Autodesk Inventor part; units mm, degrees
(part 9 of 13)
  line L3844 (34.289, 23.3701) -> (34.289, 23.1233) construction
  line L3845 (34.289, 23.1233) -> (34.4891, 22.9231) construction
  line L3846 (34.4891, 22.9231) -> (34.7358, 22.9231) construction
  spline S1207 degree 3 poles (34.7358, 22.9231) (34.9826, 22.9231) (35.1829, 23.1233) (35.1829, 23.3701) knots 0 0 0 0 1 1 1 1
  line L3847 (34.7358, 22.9231) -> (34.9826, 22.9231) construction
  line L3848 (34.9826, 22.9231) -> (35.1829, 23.1233) construction
  line L3849 (35.1829, 23.1233) -> (35.1829, 23.3701) construction
  spline S1208 degree 3 poles (35.1829, 25.9242) (35.1829, 26.171) (34.9826, 26.3711) (34.7358, 26.3711) knots 0 0 0 0 1 1 1 1
  line L3850 (35.1829, 25.9242) -> (35.1829, 26.171) construction
  line L3851 (35.1829, 26.171) -> (34.9826, 26.3711) construction
  line L3852 (34.9826, 26.3711) -> (34.7358, 26.3711) construction
  spline S1209 degree 3 poles (34.7358, 26.3711) (34.4891, 26.3711) (34.289, 26.171) (34.289, 25.9242) knots 0 0 0 0 1 1 1 1
  line L3853 (34.7358, 26.3711) -> (34.4891, 26.3711) construction
  line L3854 (34.4891, 26.3711) -> (34.289, 26.171) construction
  line L3855 (34.289, 26.171) -> (34.289, 25.9242) construction
  spline S1210 degree 3 poles (34.289, 25.9242) (34.289, 25.6775) (34.4891, 25.4772) (34.7358, 25.4772) knots 0 0 0 0 1 1 1 1
  line L3856 (34.289, 25.9242) -> (34.289, 25.6775) construction
  line L3857 (34.289, 25.6775) -> (34.4891, 25.4772) construction
  line L3858 (34.4891, 25.4772) -> (34.7358, 25.4772) construction
  spline S1211 degree 3 poles (34.7358, 25.4772) (34.9826, 25.4772) (35.1829, 25.6775) (35.1829, 25.9242) knots 0 0 0 0 1 1 1 1
  line L3859 (34.7358, 25.4772) -> (34.9826, 25.4772) construction
  line L3860 (34.9826, 25.4772) -> (35.1829, 25.6775) construction
  line L3861 (35.1829, 25.6775) -> (35.1829, 25.9242) construction
  spline S1212 degree 3 poles (35.1829, 28.4784) (35.1829, 28.7251) (34.9826, 28.9252) (34.7358, 28.9252) knots 0 0 0 0 1 1 1 1
  line L3862 (35.1829, 28.4784) -> (35.1829, 28.7251) construction
  line L3863 (35.1829, 28.7251) -> (34.9826, 28.9252) construction
  line L3864 (34.9826, 28.9252) -> (34.7358, 28.9252) construction
  spline S1213 degree 3 poles (34.7358, 28.9252) (34.4891, 28.9252) (34.289, 28.7251) (34.289, 28.4784) knots 0 0 0 0 1 1 1 1
  line L3865 (34.7358, 28.9252) -> (34.4891, 28.9252) construction
  line L3866 (34.4891, 28.9252) -> (34.289, 28.7251) construction
  line L3867 (34.289, 28.7251) -> (34.289, 28.4784) construction
  spline S1214 degree 3 poles (34.289, 28.4784) (34.289, 28.2316) (34.4891, 28.0313) (34.7358, 28.0313) knots 0 0 0 0 1 1 1 1
  line L3868 (34.289, 28.4784) -> (34.289, 28.2316) construction
  line L3869 (34.289, 28.2316) -> (34.4891, 28.0313) construction
  line L3870 (34.4891, 28.0313) -> (34.7358, 28.0313) construction
  spline S1215 degree 3 poles (34.7358, 28.0313) (34.9826, 28.0313) (35.1829, 28.2316) (35.1829, 28.4784) knots 0 0 0 0 1 1 1 1
  line L3871 (34.7358, 28.0313) -> (34.9826, 28.0313) construction
  line L3872 (34.9826, 28.0313) -> (35.1829, 28.2316) construction
  line L3873 (35.1829, 28.2316) -> (35.1829, 28.4784) construction
  spline S1216 degree 3 poles (35.1829, 31.0325) (35.1829, 31.2793) (34.9826, 31.4793) (34.7358, 31.4793) knots 0 0 0 0 1 1 1 1
  line L3874 (35.1829, 31.0325) -> (35.1829, 31.2793) construction
  line L3875 (35.1829, 31.2793) -> (34.9826, 31.4793) construction
  line L3876 (34.9826, 31.4793) -> (34.7358, 31.4793) construction
  spline S1217 degree 3 poles (34.7358, 31.4793) (34.4891, 31.4793) (34.289, 31.2793) (34.289, 31.0325) knots 0 0 0 0 1 1 1 1
  line L3877 (34.7358, 31.4793) -> (34.4891, 31.4793) construction
  line L3878 (34.4891, 31.4793) -> (34.289, 31.2793) construction
  line L3879 (34.289, 31.2793) -> (34.289, 31.0325) construction
  spline S1218 degree 3 poles (34.289, 31.0325) (34.289, 30.7857) (34.4891, 30.5854) (34.7358, 30.5854) knots 0 0 0 0 1 1 1 1
  line L3880 (34.289, 31.0325) -> (34.289, 30.7857) construction
  line L3881 (34.289, 30.7857) -> (34.4891, 30.5854) construction
  line L3882 (34.4891, 30.5854) -> (34.7358, 30.5854) construction
  spline S1219 degree 3 poles (34.7358, 30.5854) (34.9826, 30.5854) (35.1829, 30.7857) (35.1829, 31.0325) knots 0 0 0 0 1 1 1 1
  line L3883 (34.7358, 30.5854) -> (34.9826, 30.5854) construction
  line L3884 (34.9826, 30.5854) -> (35.1829, 30.7857) construction
  line L3885 (35.1829, 30.7857) -> (35.1829, 31.0325) construction
  spline S1220 degree 3 poles (37.737, 20.816) (37.737, 21.0628) (37.5369, 21.2629) (37.29, 21.2629) knots 0 0 0 0 1 1 1 1
  line L3886 (37.737, 20.816) -> (37.737, 21.0628) construction
  line L3887 (37.737, 21.0628) -> (37.5369, 21.2629) construction
  line L3888 (37.5369, 21.2629) -> (37.29, 21.2629) construction
  spline S1221 degree 3 poles (37.29, 21.2629) (37.0431, 21.2629) (36.843, 21.0628) (36.843, 20.816) knots 0 0 0 0 1 1 1 1
  line L3889 (37.29, 21.2629) -> (37.0431, 21.2629) construction
  line L3890 (37.0431, 21.2629) -> (36.843, 21.0628) construction
  line L3891 (36.843, 21.0628) -> (36.843, 20.816) construction
  spline S1222 degree 3 poles (36.843, 20.816) (36.843, 20.5692) (37.0431, 20.369) (37.29, 20.369) knots 0 0 0 0 1 1 1 1
  line L3892 (36.843, 20.816) -> (36.843, 20.5692) construction
  line L3893 (36.843, 20.5692) -> (37.0431, 20.369) construction
  line L3894 (37.0431, 20.369) -> (37.29, 20.369) construction
  spline S1223 degree 3 poles (37.29, 20.369) (37.5369, 20.369) (37.737, 20.5692) (37.737, 20.816) knots 0 0 0 0 1 1 1 1
  line L3895 (37.29, 20.369) -> (37.5369, 20.369) construction
  line L3896 (37.5369, 20.369) -> (37.737, 20.5692) construction
  line L3897 (37.737, 20.5692) -> (37.737, 20.816) construction
  spline S1224 degree 3 poles (37.737, 23.3701) (37.737, 23.6169) (37.5369, 23.817) (37.29, 23.817) knots 0 0 0 0 1 1 1 1
  line L3898 (37.737, 23.3701) -> (37.737, 23.6169) construction
  line L3899 (37.737, 23.6169) -> (37.5369, 23.817) construction
  line L3900 (37.5369, 23.817) -> (37.29, 23.817) construction
  spline S1225 degree 3 poles (37.29, 23.817) (37.0431, 23.817) (36.843, 23.6169) (36.843, 23.3701) knots 0 0 0 0 1 1 1 1
  line L3901 (37.29, 23.817) -> (37.0431, 23.817) construction
  line L3902 (37.0431, 23.817) -> (36.843, 23.6169) construction
  line L3903 (36.843, 23.6169) -> (36.843, 23.3701) construction
  spline S1226 degree 3 poles (36.843, 23.3701) (36.843, 23.1233) (37.0431, 22.9231) (37.29, 22.9231) knots 0 0 0 0 1 1 1 1
  line L3904 (36.843, 23.3701) -> (36.843, 23.1233) construction
  line L3905 (36.843, 23.1233) -> (37.0431, 22.9231) construction
  line L3906 (37.0431, 22.9231) -> (37.29, 22.9231) construction
  spline S1227 degree 3 poles (37.29, 22.9231) (37.5369, 22.9231) (37.737, 23.1233) (37.737, 23.3701) knots 0 0 0 0 1 1 1 1
  line L3907 (37.29, 22.9231) -> (37.5369, 22.9231) construction
  line L3908 (37.5369, 22.9231) -> (37.737, 23.1233) construction
  line L3909 (37.737, 23.1233) -> (37.737, 23.3701) construction
  spline S1228 degree 3 poles (37.737, 25.9242) (37.737, 26.171) (37.5369, 26.3711) (37.29, 26.3711) knots 0 0 0 0 1 1 1 1
  line L3910 (37.737, 25.9242) -> (37.737, 26.171) construction
  line L3911 (37.737, 26.171) -> (37.5369, 26.3711) construction
  line L3912 (37.5369, 26.3711) -> (37.29, 26.3711) construction
  spline S1229 degree 3 poles (37.29, 26.3711) (37.0431, 26.3711) (36.843, 26.171) (36.843, 25.9242) knots 0 0 0 0 1 1 1 1
  line L3913 (37.29, 26.3711) -> (37.0431, 26.3711) construction
  line L3914 (37.0431, 26.3711) -> (36.843, 26.171) construction
  line L3915 (36.843, 26.171) -> (36.843, 25.9242) construction
  spline S1230 degree 3 poles (36.843, 25.9242) (36.843, 25.6775) (37.0431, 25.4772) (37.29, 25.4772) knots 0 0 0 0 1 1 1 1
  line L3916 (36.843, 25.9242) -> (36.843, 25.6775) construction
  line L3917 (36.843, 25.6775) -> (37.0431, 25.4772) construction
  line L3918 (37.0431, 25.4772) -> (37.29, 25.4772) construction
  spline S1231 degree 3 poles (37.29, 25.4772) (37.5369, 25.4772) (37.737, 25.6775) (37.737, 25.9242) knots 0 0 0 0 1 1 1 1
  line L3919 (37.29, 25.4772) -> (37.5369, 25.4772) construction
  line L3920 (37.5369, 25.4772) -> (37.737, 25.6775) construction
  line L3921 (37.737, 25.6775) -> (37.737, 25.9242) construction
  spline S1232 degree 3 poles (37.737, 28.4784) (37.737, 28.7251) (37.5369, 28.9252) (37.29, 28.9252) knots 0 0 0 0 1 1 1 1
  line L3922 (37.737, 28.4784) -> (37.737, 28.7251) construction
  line L3923 (37.737, 28.7251) -> (37.5369, 28.9252) construction
  line L3924 (37.5369, 28.9252) -> (37.29, 28.9252) construction
  spline S1233 degree 3 poles (37.29, 28.9252) (37.0431, 28.9252) (36.843, 28.7251) (36.843, 28.4784) knots 0 0 0 0 1 1 1 1
  line L3925 (37.29, 28.9252) -> (37.0431, 28.9252) construction
  line L3926 (37.0431, 28.9252) -> (36.843, 28.7251) construction
  line L3927 (36.843, 28.7251) -> (36.843, 28.4784) construction
  spline S1234 degree 3 poles (36.843, 28.4784) (36.843, 28.2316) (37.0431, 28.0313) (37.29, 28.0313) knots 0 0 0 0 1 1 1 1
  line L3928 (36.843, 28.4784) -> (36.843, 28.2316) construction
  line L3929 (36.843, 28.2316) -> (37.0431, 28.0313) construction
  line L3930 (37.0431, 28.0313) -> (37.29, 28.0313) construction
  spline S1235 degree 3 poles (37.29, 28.0313) (37.5369, 28.0313) (37.737, 28.2316) (37.737, 28.4784) knots 0 0 0 0 1 1 1 1
  line L3931 (37.29, 28.0313) -> (37.5369, 28.0313) construction
  line L3932 (37.5369, 28.0313) -> (37.737, 28.2316) construction
  line L3933 (37.737, 28.2316) -> (37.737, 28.4784) construction
  spline S1236 degree 3 poles (37.737, 31.0325) (37.737, 31.2793) (37.5369, 31.4793) (37.29, 31.4793) knots 0 0 0 0 1 1 1 1
  line L3934 (37.737, 31.0325) -> (37.737, 31.2793) construction
  line L3935 (37.737, 31.2793) -> (37.5369, 31.4793) construction
  line L3936 (37.5369, 31.4793) -> (37.29, 31.4793) construction
  spline S1237 degree 3 poles (37.29, 31.4793) (37.0431, 31.4793) (36.843, 31.2793) (36.843, 31.0325) knots 0 0 0 0 1 1 1 1
  line L3937 (37.29, 31.4793) -> (37.0431, 31.4793) construction
  line L3938 (37.0431, 31.4793) -> (36.843, 31.2793) construction
  line L3939 (36.843, 31.2793) -> (36.843, 31.0325) construction
  spline S1238 degree 3 poles (36.843, 31.0325) (36.843, 30.7857) (37.0431, 30.5854) (37.29, 30.5854) knots 0 0 0 0 1 1 1 1
  line L3940 (36.843, 31.0325) -> (36.843, 30.7857) construction
  line L3941 (36.843, 30.7857) -> (37.0431, 30.5854) construction
  line L3942 (37.0431, 30.5854) -> (37.29, 30.5854) construction
  spline S1239 degree 3 poles (37.29, 30.5854) (37.5369, 30.5854) (37.737, 30.7857) (37.737, 31.0325) knots 0 0 0 0 1 1 1 1
  line L3943 (37.29, 30.5854) -> (37.5369, 30.5854) construction
  line L3944 (37.5369, 30.5854) -> (37.737, 30.7857) construction
  line L3945 (37.737, 30.7857) -> (37.737, 31.0325) construction
  spline S1240 degree 3 poles (45.3993, 0.3832) (45.3993, 0.6299) (45.1992, 0.83) (44.9523, 0.83) knots 0 0 0 0 1 1 1 1
  line L3946 (45.3993, 0.3832) -> (45.3993, 0.6299) construction
  line L3947 (45.3993, 0.6299) -> (45.1992, 0.83) construction
  line L3948 (45.1992, 0.83) -> (44.9523, 0.83) construction
  spline S1241 degree 3 poles (44.9523, 0.83) (44.7054, 0.83) (44.5054, 0.6299) (44.5054, 0.3832) knots 0 0 0 0 1 1 1 1
  line L3949 (44.9523, 0.83) -> (44.7054, 0.83) construction
  line L3950 (44.7054, 0.83) -> (44.5054, 0.6299) construction
  line L3951 (44.5054, 0.6299) -> (44.5054, 0.3832) construction
  spline S1242 degree 3 poles (44.5054, 0.3832) (44.5054, 0.1364) (44.7054, -0.0639) (44.9523, -0.0639) knots 0 0 0 0 1 1 1 1
  line L3952 (44.5054, 0.3832) -> (44.5054, 0.1364) construction
  line L3953 (44.5054, 0.1364) -> (44.7054, -0.0639) construction
  line L3954 (44.7054, -0.0639) -> (44.9523, -0.0639) construction
  spline S1243 degree 3 poles (44.9523, -0.0639) (45.1992, -0.0639) (45.3993, 0.1364) (45.3993, 0.3832) knots 0 0 0 0 1 1 1 1
  line L3955 (44.9523, -0.0639) -> (45.1992, -0.0639) construction
  line L3956 (45.1992, -0.0639) -> (45.3993, 0.1364) construction
  line L3957 (45.3993, 0.1364) -> (45.3993, 0.3832) construction
  spline S1244 degree 3 poles (47.9534, 0.3832) (47.9534, 0.6299) (47.7533, 0.83) (47.5064, 0.83) knots 0 0 0 0 1 1 1 1
  line L3958 (47.9534, 0.3832) -> (47.9534, 0.6299) construction
  line L3959 (47.9534, 0.6299) -> (47.7533, 0.83) construction
  line L3960 (47.7533, 0.83) -> (47.5064, 0.83) construction
  spline S1245 degree 3 poles (47.5064, 0.83) (47.2595, 0.83) (47.0595, 0.6299) (47.0595, 0.3832) knots 0 0 0 0 1 1 1 1
  line L3961 (47.5064, 0.83) -> (47.2595, 0.83) construction
  line L3962 (47.2595, 0.83) -> (47.0595, 0.6299) construction
  line L3963 (47.0595, 0.6299) -> (47.0595, 0.3832) construction
  spline S1246 degree 3 poles (47.0595, 0.3832) (47.0595, 0.1364) (47.2595, -0.0639) (47.5064, -0.0639) knots 0 0 0 0 1 1 1 1
  line L3964 (47.0595, 0.3832) -> (47.0595, 0.1364) construction
  line L3965 (47.0595, 0.1364) -> (47.2595, -0.0639) construction
  line L3966 (47.2595, -0.0639) -> (47.5064, -0.0639) construction
  spline S1247 degree 3 poles (47.5064, -0.0639) (47.7533, -0.0639) (47.9534, 0.1364) (47.9534, 0.3832) knots 0 0 0 0 1 1 1 1
  line L3967 (47.5064, -0.0639) -> (47.7533, -0.0639) construction
  line L3968 (47.7533, -0.0639) -> (47.9534, 0.1364) construction
  line L3969 (47.9534, 0.1364) -> (47.9534, 0.3832) construction
  spline S1248 degree 3 poles (46.6763, 9.7057) (46.6763, 10.5872) (45.9615, 11.302) (45.08, 11.302) knots 0 0 0 0 1 1 1 1
  line L3970 (46.6763, 9.7057) -> (46.6763, 10.5872) construction
  line L3971 (46.6763, 10.5872) -> (45.9615, 11.302) construction
  line L3972 (45.9615, 11.302) -> (45.08, 11.302) construction
  spline S1249 degree 3 poles (45.08, 11.302) (44.1985, 11.302) (43.4837, 10.5872) (43.4837, 9.7057) knots 0 0 0 0 1 1 1 1
  line L3973 (45.08, 11.302) -> (44.1985, 11.302) construction
  line L3974 (44.1985, 11.302) -> (43.4837, 10.5872) construction
  line L3975 (43.4837, 10.5872) -> (43.4837, 9.7057) construction
  spline S1250 degree 3 poles (43.4837, 9.7057) (43.4837, 8.8241) (44.1985, 8.1094) (45.08, 8.1094) knots 0 0 0 0 1 1 1 1
  line L3976 (43.4837, 9.7057) -> (43.4837, 8.8241) construction
  line L3977 (43.4837, 8.8241) -> (44.1985, 8.1094) construction
  line L3978 (44.1985, 8.1094) -> (45.08, 8.1094) construction
  spline S1251 degree 3 poles (45.08, 8.1094) (45.9615, 8.1094) (46.6763, 8.8241) (46.6763, 9.7057) knots 0 0 0 0 1 1 1 1
  line L3979 (45.08, 8.1094) -> (45.9615, 8.1094) construction
  line L3980 (45.9615, 8.1094) -> (46.6763, 8.8241) construction
  line L3981 (46.6763, 8.8241) -> (46.6763, 9.7057) construction
  spline S1252 degree 3 poles (52.8701, 9.7057) (52.8701, 10.4814) (52.2411, 11.1103) (51.4653, 11.1103) knots 0 0 0 0 1 1 1 1
  line L3982 (52.8701, 9.7057) -> (52.8701, 10.4814) construction
  line L3983 (52.8701, 10.4814) -> (52.2411, 11.1103) construction
  line L3984 (52.2411, 11.1103) -> (51.4653, 11.1103) construction
  spline S1253 degree 3 poles (51.4653, 11.1103) (50.6895, 11.1103) (50.0605, 10.4814) (50.0605, 9.7057) knots 0 0 0 0 1 1 1 1
  line L3985 (51.4653, 11.1103) -> (50.6895, 11.1103) construction
  line L3986 (50.6895, 11.1103) -> (50.0605, 10.4814) construction
  line L3987 (50.0605, 10.4814) -> (50.0605, 9.7057) construction
  spline S1254 degree 3 poles (50.0605, 9.7057) (50.0605, 8.9299) (50.6895, 8.3009) (51.4653, 8.3009) knots 0 0 0 0 1 1 1 1
  line L3988 (50.0605, 9.7057) -> (50.0605, 8.9299) construction
  line L3989 (50.0605, 8.9299) -> (50.6895, 8.3009) construction
  line L3990 (50.6895, 8.3009) -> (51.4653, 8.3009) construction
  spline S1255 degree 3 poles (51.4653, 8.3009) (52.2411, 8.3009) (52.8701, 8.9299) (52.8701, 9.7057) knots 0 0 0 0 1 1 1 1
  line L3991 (51.4653, 8.3009) -> (52.2411, 8.3009) construction
  line L3992 (52.2411, 8.3009) -> (52.8701, 8.9299) construction
  line L3993 (52.8701, 8.9299) -> (52.8701, 9.7057) construction
  spline S1256 degree 3 poles (49.6774, 14.303) (49.6774, 15.0787) (49.0485, 15.7078) (48.2727, 15.7078) knots 0 0 0 0 1 1 1 1
  line L3994 (49.6774, 14.303) -> (49.6774, 15.0787) construction
  line L3995 (49.6774, 15.0787) -> (49.0485, 15.7078) construction
  line L3996 (49.0485, 15.7078) -> (48.2727, 15.7078) construction
  spline S1257 degree 3 poles (48.2727, 15.7078) (47.4969, 15.7078) (46.8679, 15.0787) (46.8679, 14.303) knots 0 0 0 0 1 1 1 1
  line L3997 (48.2727, 15.7078) -> (47.4969, 15.7078) construction
  line L3998 (47.4969, 15.7078) -> (46.8679, 15.0787) construction
  line L3999 (46.8679, 15.0787) -> (46.8679, 14.303) construction
  spline S1258 degree 3 poles (46.8679, 14.303) (46.8679, 13.5273) (47.4969, 12.8983) (48.2727, 12.8983) knots 0 0 0 0 1 1 1 1
  line L4000 (46.8679, 14.303) -> (46.8679, 13.5273) construction
  line L4001 (46.8679, 13.5273) -> (47.4969, 12.8983) construction
  line L4002 (47.4969, 12.8983) -> (48.2727, 12.8983) construction
  spline S1259 degree 3 poles (48.2727, 12.8983) (49.0485, 12.8983) (49.6774, 13.5273) (49.6774, 14.303) knots 0 0 0 0 1 1 1 1
  line L4003 (48.2727, 12.8983) -> (49.0485, 12.8983) construction
  line L4004 (49.0485, 12.8983) -> (49.6774, 13.5273) construction
  line L4005 (49.6774, 13.5273) -> (49.6774, 14.303) construction
  spline S1260 degree 3 poles (9.6418, 0.3832) (9.6418, 0.6299) (9.4415, 0.83) (9.1948, 0.83) knots 0 0 0 0 1 1 1 1
  line L4006 (9.6418, 0.3832) -> (9.6418, 0.6299) construction
  line L4007 (9.6418, 0.6299) -> (9.4415, 0.83) construction
  line L4008 (9.4415, 0.83) -> (9.1948, 0.83) construction
  spline S1261 degree 3 poles (9.1948, 0.83) (8.948, 0.83) (8.7479, 0.6299) (8.7479, 0.3832) knots 0 0 0 0 1 1 1 1
  line L4009 (9.1948, 0.83) -> (8.948, 0.83) construction
  line L4010 (8.948, 0.83) -> (8.7479, 0.6299) construction
  line L4011 (8.7479, 0.6299) -> (8.7479, 0.3832) construction
  spline S1262 degree 3 poles (8.7479, 0.3832) (8.7479, 0.1364) (8.948, -0.0639) (9.1948, -0.0639) knots 0 0 0 0 1 1 1 1
  line L4012 (8.7479, 0.3832) -> (8.7479, 0.1364) construction
  line L4013 (8.7479, 0.1364) -> (8.948, -0.0639) construction
  line L4014 (8.948, -0.0639) -> (9.1948, -0.0639) construction
  spline S1263 degree 3 poles (9.1948, -0.0639) (9.4415, -0.0639) (9.6418, 0.1364) (9.6418, 0.3832) knots 0 0 0 0 1 1 1 1
  line L4015 (9.1948, -0.0639) -> (9.4415, -0.0639) construction
  line L4016 (9.4415, -0.0639) -> (9.6418, 0.1364) construction
  line L4017 (9.6418, 0.1364) -> (9.6418, 0.3832) construction
  spline S1264 degree 3 poles (12.1959, 0.3832) (12.1959, 0.6299) (11.9957, 0.83) (11.7489, 0.83) knots 0 0 0 0 1 1 1 1
  line L4018 (12.1959, 0.3832) -> (12.1959, 0.6299) construction
  line L4019 (12.1959, 0.6299) -> (11.9957, 0.83) construction
  line L4020 (11.9957, 0.83) -> (11.7489, 0.83) construction
  spline S1265 degree 3 poles (11.7489, 0.83) (11.5021, 0.83) (11.302, 0.6299) (11.302, 0.3832) knots 0 0 0 0 1 1 1 1
  line L4021 (11.7489, 0.83) -> (11.5021, 0.83) construction
  line L4022 (11.5021, 0.83) -> (11.302, 0.6299) construction
  line L4023 (11.302, 0.6299) -> (11.302, 0.3832) construction
  spline S1266 degree 3 poles (11.302, 0.3832) (11.302, 0.1364) (11.5021, -0.0639) (11.7489, -0.0639) knots 0 0 0 0 1 1 1 1
  line L4024 (11.302, 0.3832) -> (11.302, 0.1364) construction
  line L4025 (11.302, 0.1364) -> (11.5021, -0.0639) construction
  line L4026 (11.5021, -0.0639) -> (11.7489, -0.0639) construction
  spline S1267 degree 3 poles (11.7489, -0.0639) (11.9957, -0.0639) (12.1959, 0.1364) (12.1959, 0.3832) knots 0 0 0 0 1 1 1 1
  line L4027 (11.7489, -0.0639) -> (11.9957, -0.0639) construction
  line L4028 (11.9957, -0.0639) -> (12.1959, 0.1364) construction
  line L4029 (12.1959, 0.1364) -> (12.1959, 0.3832) construction
  spline S1268 degree 3 poles (14.75, 0.3832) (14.75, 0.6299) (14.5498, 0.83) (14.303, 0.83) knots 0 0 0 0 1 1 1 1
  line L4030 (14.75, 0.3832) -> (14.75, 0.6299) construction
  line L4031 (14.75, 0.6299) -> (14.5498, 0.83) construction
  line L4032 (14.5498, 0.83) -> (14.303, 0.83) construction
  spline S1269 degree 3 poles (14.303, 0.83) (14.0562, 0.83) (13.8561, 0.6299) (13.8561, 0.3832) knots 0 0 0 0 1 1 1 1
  line L4033 (14.303, 0.83) -> (14.0562, 0.83) construction
  line L4034 (14.0562, 0.83) -> (13.8561, 0.6299) construction
  line L4035 (13.8561, 0.6299) -> (13.8561, 0.3832) construction
  spline S1270 degree 3 poles (13.8561, 0.3832) (13.8561, 0.1364) (14.0562, -0.0639) (14.303, -0.0639) knots 0 0 0 0 1 1 1 1
  line L4036 (13.8561, 0.3832) -> (13.8561, 0.1364) construction
  line L4037 (13.8561, 0.1364) -> (14.0562, -0.0639) construction
  line L4038 (14.0562, -0.0639) -> (14.303, -0.0639) construction
  spline S1271 degree 3 poles (14.303, -0.0639) (14.5498, -0.0639) (14.75, 0.1364) (14.75, 0.3832) knots 0 0 0 0 1 1 1 1
  line L4039 (14.303, -0.0639) -> (14.5498, -0.0639) construction
  line L4040 (14.5498, -0.0639) -> (14.75, 0.1364) construction
  line L4041 (14.75, 0.1364) -> (14.75, 0.3832) construction
  spline S1272 degree 3 poles (17.3041, 0.3832) (17.3041, 0.6299) (17.1039, 0.83) (16.8571, 0.83) knots 0 0 0 0 1 1 1 1
  line L4042 (17.3041, 0.3832) -> (17.3041, 0.6299) construction
  line L4043 (17.3041, 0.6299) -> (17.1039, 0.83) construction
  line L4044 (17.1039, 0.83) -> (16.8571, 0.83) construction
  spline S1273 degree 3 poles (16.8571, 0.83) (16.6103, 0.83) (16.4102, 0.6299) (16.4102, 0.3832) knots 0 0 0 0 1 1 1 1
  line L4045 (16.8571, 0.83) -> (16.6103, 0.83) construction
  line L4046 (16.6103, 0.83) -> (16.4102, 0.6299) construction
  line L4047 (16.4102, 0.6299) -> (16.4102, 0.3832) construction
  spline S1274 degree 3 poles (16.4102, 0.3832) (16.4102, 0.1364) (16.6103, -0.0639) (16.8571, -0.0639) knots 0 0 0 0 1 1 1 1
  line L4048 (16.4102, 0.3832) -> (16.4102, 0.1364) construction
  line L4049 (16.4102, 0.1364) -> (16.6103, -0.0639) construction
  line L4050 (16.6103, -0.0639) -> (16.8571, -0.0639) construction
  spline S1275 degree 3 poles (16.8571, -0.0639) (17.1039, -0.0639) (17.3041, 0.1364) (17.3041, 0.3832) knots 0 0 0 0 1 1 1 1
  line L4051 (16.8571, -0.0639) -> (17.1039, -0.0639) construction
  line L4052 (17.1039, -0.0639) -> (17.3041, 0.1364) construction
  line L4053 (17.3041, 0.1364) -> (17.3041, 0.3832) construction
  spline S1276 degree 3 poles (17.3041, 2.9373) (17.3041, 3.1841) (17.1039, 3.3841) (16.8571, 3.3841) knots 0 0 0 0 1 1 1 1
  line L4054 (17.3041, 2.9373) -> (17.3041, 3.1841) construction
  line L4055 (17.3041, 3.1841) -> (17.1039, 3.3841) construction
  line L4056 (17.1039, 3.3841) -> (16.8571, 3.3841) construction
  spline S1277 degree 3 poles (16.8571, 3.3841) (16.6103, 3.3841) (16.4102, 3.1841) (16.4102, 2.9373) knots 0 0 0 0 1 1 1 1
  line L4057 (16.8571, 3.3841) -> (16.6103, 3.3841) construction
  line L4058 (16.6103, 3.3841) -> (16.4102, 3.1841) construction
  line L4059 (16.4102, 3.1841) -> (16.4102, 2.9373) construction
  spline S1278 degree 3 poles (16.4102, 2.9373) (16.4102, 2.6905) (16.6103, 2.4902) (16.8571, 2.4902) knots 0 0 0 0 1 1 1 1
  line L4060 (16.4102, 2.9373) -> (16.4102, 2.6905) construction
  line L4061 (16.4102, 2.6905) -> (16.6103, 2.4902) construction
  line L4062 (16.6103, 2.4902) -> (16.8571, 2.4902) construction
  spline S1279 degree 3 poles (16.8571, 2.4902) (17.1039, 2.4902) (17.3041, 2.6905) (17.3041, 2.9373) knots 0 0 0 0 1 1 1 1
  line L4063 (16.8571, 2.4902) -> (17.1039, 2.4902) construction
  line L4064 (17.1039, 2.4902) -> (17.3041, 2.6905) construction
  line L4065 (17.3041, 2.6905) -> (17.3041, 2.9373) construction
  spline S1280 degree 3 poles (19.8582, 2.9373) (19.8582, 3.1841) (19.658, 3.3841) (19.4112, 3.3841) knots 0 0 0 0 1 1 1 1
  line L4066 (19.8582, 2.9373) -> (19.8582, 3.1841) construction
  line L4067 (19.8582, 3.1841) -> (19.658, 3.3841) construction
  line L4068 (19.658, 3.3841) -> (19.4112, 3.3841) construction
  spline S1281 degree 3 poles (19.4112, 3.3841) (19.1644, 3.3841) (18.9643, 3.1841) (18.9643, 2.9373) knots 0 0 0 0 1 1 1 1
  line L4069 (19.4112, 3.3841) -> (19.1644, 3.3841) construction
  line L4070 (19.1644, 3.3841) -> (18.9643, 3.1841) construction
  line L4071 (18.9643, 3.1841) -> (18.9643, 2.9373) construction
  spline S1282 degree 3 poles (18.9643, 2.9373) (18.9643, 2.6905) (19.1644, 2.4902) (19.4112, 2.4902) knots 0 0 0 0 1 1 1 1
  line L4072 (18.9643, 2.9373) -> (18.9643, 2.6905) construction
  line L4073 (18.9643, 2.6905) -> (19.1644, 2.4902) construction
  line L4074 (19.1644, 2.4902) -> (19.4112, 2.4902) construction
  spline S1283 degree 3 poles (19.4112, 2.4902) (19.658, 2.4902) (19.8582, 2.6905) (19.8582, 2.9373) knots 0 0 0 0 1 1 1 1
  line L4075 (19.4112, 2.4902) -> (19.658, 2.4902) construction
  line L4076 (19.658, 2.4902) -> (19.8582, 2.6905) construction
  line L4077 (19.8582, 2.6905) -> (19.8582, 2.9373) construction
  spline S1284 degree 3 poles (26.2435, 0.3832) (26.2435, 0.6299) (26.0433, 0.83) (25.7965, 0.83) knots 0 0 0 0 1 1 1 1
  line L4078 (26.2435, 0.3832) -> (26.2435, 0.6299) construction
  line L4079 (26.2435, 0.6299) -> (26.0433, 0.83) construction
  line L4080 (26.0433, 0.83) -> (25.7965, 0.83) construction
  spline S1285 degree 3 poles (25.7965, 0.83) (25.5497, 0.83) (25.3496, 0.6299) (25.3496, 0.3832) knots 0 0 0 0 1 1 1 1
  line L4081 (25.7965, 0.83) -> (25.5497, 0.83) construction
  line L4082 (25.5497, 0.83) -> (25.3496, 0.6299) construction
  line L4083 (25.3496, 0.6299) -> (25.3496, 0.3832) construction
  spline S1286 degree 3 poles (25.3496, 0.3832) (25.3496, 0.1364) (25.5497, -0.0639) (25.7965, -0.0639) knots 0 0 0 0 1 1 1 1
  line L4084 (25.3496, 0.3832) -> (25.3496, 0.1364) construction
  line L4085 (25.3496, 0.1364) -> (25.5497, -0.0639) construction
  line L4086 (25.5497, -0.0639) -> (25.7965, -0.0639) construction
  spline S1287 degree 3 poles (25.7965, -0.0639) (26.0433, -0.0639) (26.2435, 0.1364) (26.2435, 0.3832) knots 0 0 0 0 1 1 1 1
  line L4087 (25.7965, -0.0639) -> (26.0433, -0.0639) construction
  line L4088 (26.0433, -0.0639) -> (26.2435, 0.1364) construction
  line L4089 (26.2435, 0.1364) -> (26.2435, 0.3832) construction
  spline S1288 degree 3 poles (23.6894, 0.3832) (23.6894, 0.6299) (23.4891, 0.83) (23.2424, 0.83) knots 0 0 0 0 1 1 1 1
  line L4090 (23.6894, 0.3832) -> (23.6894, 0.6299) construction
  line L4091 (23.6894, 0.6299) -> (23.4891, 0.83) construction
  line L4092 (23.4891, 0.83) -> (23.2424, 0.83) construction
  spline S1289 degree 3 poles (23.2424, 0.83) (22.9956, 0.83) (22.7955, 0.6299) (22.7955, 0.3832) knots 0 0 0 0 1 1 1 1
  line L4093 (23.2424, 0.83) -> (22.9956, 0.83) construction
  line L4094 (22.9956, 0.83) -> (22.7955, 0.6299) construction
  line L4095 (22.7955, 0.6299) -> (22.7955, 0.3832) construction
  spline S1290 degree 3 poles (22.7955, 0.3832) (22.7955, 0.1364) (22.9956, -0.0639) (23.2424, -0.0639) knots 0 0 0 0 1 1 1 1
  line L4096 (22.7955, 0.3832) -> (22.7955, 0.1364) construction
  line L4097 (22.7955, 0.1364) -> (22.9956, -0.0639) construction
  line L4098 (22.9956, -0.0639) -> (23.2424, -0.0639) construction
  spline S1291 degree 3 poles (23.2424, -0.0639) (23.4891, -0.0639) (23.6894, 0.1364) (23.6894, 0.3832) knots 0 0 0 0 1 1 1 1
  line L4099 (23.2424, -0.0639) -> (23.4891, -0.0639) construction
  line L4100 (23.4891, -0.0639) -> (23.6894, 0.1364) construction
  line L4101 (23.6894, 0.1364) -> (23.6894, 0.3832) construction
  spline S1292 degree 3 poles (21.1353, 0.3832) (21.1353, 0.6299) (20.935, 0.83) (20.6882, 0.83) knots 0 0 0 0 1 1 1 1
  line L4102 (21.1353, 0.3832) -> (21.1353, 0.6299) construction
  line L4103 (21.1353, 0.6299) -> (20.935, 0.83) construction
  line L4104 (20.935, 0.83) -> (20.6882, 0.83) construction
  spline S1293 degree 3 poles (20.6882, 0.83) (20.4415, 0.83) (20.2414, 0.6299) (20.2414, 0.3832) knots 0 0 0 0 1 1 1 1
  line L4105 (20.6882, 0.83) -> (20.4415, 0.83) construction
  line L4106 (20.4415, 0.83) -> (20.2414, 0.6299) construction
  line L4107 (20.2414, 0.6299) -> (20.2414, 0.3832) construction
  spline S1294 degree 3 poles (20.2414, 0.3832) (20.2414, 0.1364) (20.4415, -0.0639) (20.6882, -0.0639) knots 0 0 0 0 1 1 1 1
  line L4108 (20.2414, 0.3832) -> (20.2414, 0.1364) construction
  line L4109 (20.2414, 0.1364) -> (20.4415, -0.0639) construction
  line L4110 (20.4415, -0.0639) -> (20.6882, -0.0639) construction
  spline S1295 degree 3 poles (20.6882, -0.0639) (20.935, -0.0639) (21.1353, 0.1364) (21.1353, 0.3832) knots 0 0 0 0 1 1 1 1
  line L4111 (20.6882, -0.0639) -> (20.935, -0.0639) construction
  line L4112 (20.935, -0.0639) -> (21.1353, 0.1364) construction
  line L4113 (21.1353, 0.1364) -> (21.1353, 0.3832) construction
  spline S1296 degree 3 poles (19.8582, 5.4914) (19.8582, 5.7382) (19.658, 5.9382) (19.4112, 5.9382) knots 0 0 0 0 1 1 1 1
  line L4114 (19.8582, 5.4914) -> (19.8582, 5.7382) construction
  line L4115 (19.8582, 5.7382) -> (19.658, 5.9382) construction
  line L4116 (19.658, 5.9382) -> (19.4112, 5.9382) construction
  spline S1297 degree 3 poles (19.4112, 5.9382) (19.1644, 5.9382) (18.9643, 5.7382) (18.9643, 5.4914) knots 0 0 0 0 1 1 1 1
  line L4117 (19.4112, 5.9382) -> (19.1644, 5.9382) construction
  line L4118 (19.1644, 5.9382) -> (18.9643, 5.7382) construction
  line L4119 (18.9643, 5.7382) -> (18.9643, 5.4914) construction
  spline S1298 degree 3 poles (18.9643, 5.4914) (18.9643, 5.2446) (19.1644, 5.0443) (19.4112, 5.0443) knots 0 0 0 0 1 1 1 1
  line L4120 (18.9643, 5.4914) -> (18.9643, 5.2446) construction
  line L4121 (18.9643, 5.2446) -> (19.1644, 5.0443) construction
  line L4122 (19.1644, 5.0443) -> (19.4112, 5.0443) construction
  spline S1299 degree 3 poles (19.4112, 5.0443) (19.658, 5.0443) (19.8582, 5.2446) (19.8582, 5.4914) knots 0 0 0 0 1 1 1 1
  line L4123 (19.4112, 5.0443) -> (19.658, 5.0443) construction
  line L4124 (19.658, 5.0443) -> (19.8582, 5.2446) construction
  line L4125 (19.8582, 5.2446) -> (19.8582, 5.4914) construction
  spline S1300 degree 3 poles (19.8582, 8.0455) (19.8582, 8.2923) (19.658, 8.4923) (19.4112, 8.4923) knots 0 0 0 0 1 1 1 1
  line L4126 (19.8582, 8.0455) -> (19.8582, 8.2923) construction
  line L4127 (19.8582, 8.2923) -> (19.658, 8.4923) construction
  line L4128 (19.658, 8.4923) -> (19.4112, 8.4923) construction
  spline S1301 degree 3 poles (19.4112, 8.4923) (19.1644, 8.4923) (18.9643, 8.2923) (18.9643, 8.0455) knots 0 0 0 0 1 1 1 1
  line L4129 (19.4112, 8.4923) -> (19.1644, 8.4923) construction
  line L4130 (19.1644, 8.4923) -> (18.9643, 8.2923) construction
  line L4131 (18.9643, 8.2923) -> (18.9643, 8.0455) construction
  spline S1302 degree 3 poles (18.9643, 8.0455) (18.9643, 7.7987) (19.1644, 7.5984) (19.4112, 7.5984) knots 0 0 0 0 1 1 1 1
  line L4132 (18.9643, 8.0455) -> (18.9643, 7.7987) construction
  line L4133 (18.9643, 7.7987) -> (19.1644, 7.5984) construction
  line L4134 (19.1644, 7.5984) -> (19.4112, 7.5984) construction
  spline S1303 degree 3 poles (19.4112, 7.5984) (19.658, 7.5984) (19.8582, 7.7987) (19.8582, 8.0455) knots 0 0 0 0 1 1 1 1
  line L4135 (19.4112, 7.5984) -> (19.658, 7.5984) construction
  line L4136 (19.658, 7.5984) -> (19.8582, 7.7987) construction
  line L4137 (19.8582, 7.7987) -> (19.8582, 8.0455) construction
  spline S1304 degree 3 poles (19.8582, 10.5996) (19.8582, 10.8464) (19.658, 11.0465) (19.4112, 11.0465) knots 0 0 0 0 1 1 1 1
  line L4138 (19.8582, 10.5996) -> (19.8582, 10.8464) construction
  line L4139 (19.8582, 10.8464) -> (19.658, 11.0465) construction
  line L4140 (19.658, 11.0465) -> (19.4112, 11.0465) construction
  spline S1305 degree 3 poles (19.4112, 11.0465) (19.1644, 11.0465) (18.9643, 10.8464) (18.9643, 10.5996) knots 0 0 0 0 1 1 1 1
  line L4141 (19.4112, 11.0465) -> (19.1644, 11.0465) construction
  line L4142 (19.1644, 11.0465) -> (18.9643, 10.8464) construction
  line L4143 (18.9643, 10.8464) -> (18.9643, 10.5996) construction
  spline S1306 degree 3 poles (18.9643, 10.5996) (18.9643, 10.3528) (19.1644, 10.1525) (19.4112, 10.1525) knots 0 0 0 0 1 1 1 1
  line L4144 (18.9643, 10.5996) -> (18.9643, 10.3528) construction
  line L4145 (18.9643, 10.3528) -> (19.1644, 10.1525) construction
  line L4146 (19.1644, 10.1525) -> (19.4112, 10.1525) construction
  spline S1307 degree 3 poles (19.4112, 10.1525) (19.658, 10.1525) (19.8582, 10.3528) (19.8582, 10.5996) knots 0 0 0 0 1 1 1 1
  line L4147 (19.4112, 10.1525) -> (19.658, 10.1525) construction
  line L4148 (19.658, 10.1525) -> (19.8582, 10.3528) construction
  line L4149 (19.8582, 10.3528) -> (19.8582, 10.5996) construction
  spline S1308 degree 3 poles (22.7955, 11.7489) (22.7955, 11.9957) (22.5952, 12.1959) (22.3485, 12.1959) knots 0 0 0 0 1 1 1 1
  line L4150 (22.7955, 11.7489) -> (22.7955, 11.9957) construction
  line L4151 (22.7955, 11.9957) -> (22.5952, 12.1959) construction
  line L4152 (22.5952, 12.1959) -> (22.3485, 12.1959) construction
  spline S1309 degree 3 poles (22.3485, 12.1959) (22.1017, 12.1959) (21.9014, 11.9957) (21.9014, 11.7489) knots 0 0 0 0 1 1 1 1
  line L4153 (22.3485, 12.1959) -> (22.1017, 12.1959) construction
  line L4154 (22.1017, 12.1959) -> (21.9014, 11.9957) construction
  line L4155 (21.9014, 11.9957) -> (21.9014, 11.7489) construction
  spline S1310 degree 3 poles (21.9014, 11.7489) (21.9014, 11.5021) (22.1017, 11.302) (22.3485, 11.302) knots 0 0 0 0 1 1 1 1
  line L4156 (21.9014, 11.7489) -> (21.9014, 11.5021) construction
  line L4157 (21.9014, 11.5021) -> (22.1017, 11.302) construction
  line L4158 (22.1017, 11.302) -> (22.3485, 11.302) construction
  spline S1311 degree 3 poles (22.3485, 11.302) (22.5952, 11.302) (22.7955, 11.5021) (22.7955, 11.7489) knots 0 0 0 0 1 1 1 1
  line L4159 (22.3485, 11.302) -> (22.5952, 11.302) construction
  line L4160 (22.5952, 11.302) -> (22.7955, 11.5021) construction
  line L4161 (22.7955, 11.5021) -> (22.7955, 11.7489) construction
  spline S1312 degree 3 poles (25.3496, 11.7489) (25.3496, 11.9957) (25.1494, 12.1959) (24.9026, 12.1959) knots 0 0 0 0 1 1 1 1
  line L4162 (25.3496, 11.7489) -> (25.3496, 11.9957) construction
  line L4163 (25.3496, 11.9957) -> (25.1494, 12.1959) construction
  line L4164 (25.1494, 12.1959) -> (24.9026, 12.1959) construction
  spline S1313 degree 3 poles (24.9026, 12.1959) (24.6558, 12.1959) (24.4555, 11.9957) (24.4555, 11.7489) knots 0 0 0 0 1 1 1 1
  line L4165 (24.9026, 12.1959) -> (24.6558, 12.1959) construction
  line L4166 (24.6558, 12.1959) -> (24.4555, 11.9957) construction
  line L4167 (24.4555, 11.9957) -> (24.4555, 11.7489) construction
  spline S1314 degree 3 poles (24.4555, 11.7489) (24.4555, 11.5021) (24.6558, 11.302) (24.9026, 11.302) knots 0 0 0 0 1 1 1 1
  line L4168 (24.4555, 11.7489) -> (24.4555, 11.5021) construction
  line L4169 (24.4555, 11.5021) -> (24.6558, 11.302) construction
  line L4170 (24.6558, 11.302) -> (24.9026, 11.302) construction
  spline S1315 degree 3 poles (24.9026, 11.302) (25.1494, 11.302) (25.3496, 11.5021) (25.3496, 11.7489) knots 0 0 0 0 1 1 1 1
  line L4171 (24.9026, 11.302) -> (25.1494, 11.302) construction
  line L4172 (25.1494, 11.302) -> (25.3496, 11.5021) construction
  line L4173 (25.3496, 11.5021) -> (25.3496, 11.7489) construction
  spline S1316 degree 3 poles (22.7955, 14.303) (22.7955, 14.5498) (22.5952, 14.75) (22.3485, 14.75) knots 0 0 0 0 1 1 1 1
  line L4174 (22.7955, 14.303) -> (22.7955, 14.5498) construction
  line L4175 (22.7955, 14.5498) -> (22.5952, 14.75) construction
  line L4176 (22.5952, 14.75) -> (22.3485, 14.75) construction
  spline S1317 degree 3 poles (22.3485, 14.75) (22.1017, 14.75) (21.9014, 14.5498) (21.9014, 14.303) knots 0 0 0 0 1 1 1 1
  line L4177 (22.3485, 14.75) -> (22.1017, 14.75) construction
  line L4178 (22.1017, 14.75) -> (21.9014, 14.5498) construction
  line L4179 (21.9014, 14.5498) -> (21.9014, 14.303) construction
  spline S1318 degree 3 poles (21.9014, 14.303) (21.9014, 14.0562) (22.1017, 13.8561) (22.3485, 13.8561) knots 0 0 0 0 1 1 1 1
  line L4180 (21.9014, 14.303) -> (21.9014, 14.0562) construction
  line L4181 (21.9014, 14.0562) -> (22.1017, 13.8561) construction
  line L4182 (22.1017, 13.8561) -> (22.3485, 13.8561) construction
  spline S1319 degree 3 poles (22.3485, 13.8561) (22.5952, 13.8561) (22.7955, 14.0562) (22.7955, 14.303) knots 0 0 0 0 1 1 1 1
  line L4183 (22.3485, 13.8561) -> (22.5952, 13.8561) construction
  line L4184 (22.5952, 13.8561) -> (22.7955, 14.0562) construction
  line L4185 (22.7955, 14.0562) -> (22.7955, 14.303) construction
  spline S1320 degree 3 poles (25.3496, 14.303) (25.3496, 14.5498) (25.1494, 14.75) (24.9026, 14.75) knots 0 0 0 0 1 1 1 1
  line L4186 (25.3496, 14.303) -> (25.3496, 14.5498) construction
  line L4187 (25.3496, 14.5498) -> (25.1494, 14.75) construction
  line L4188 (25.1494, 14.75) -> (24.9026, 14.75) construction
  spline S1321 degree 3 poles (24.9026, 14.75) (24.6558, 14.75) (24.4555, 14.5498) (24.4555, 14.303) knots 0 0 0 0 1 1 1 1
  line L4189 (24.9026, 14.75) -> (24.6558, 14.75) construction
  line L4190 (24.6558, 14.75) -> (24.4555, 14.5498) construction
  line L4191 (24.4555, 14.5498) -> (24.4555, 14.303) construction
  spline S1322 degree 3 poles (24.4555, 14.303) (24.4555, 14.0562) (24.6558, 13.8561) (24.9026, 13.8561) knots 0 0 0 0 1 1 1 1
  line L4192 (24.4555, 14.303) -> (24.4555, 14.0562) construction
  line L4193 (24.4555, 14.0562) -> (24.6558, 13.8561) construction
  line L4194 (24.6558, 13.8561) -> (24.9026, 13.8561) construction
  spline S1323 degree 3 poles (24.9026, 13.8561) (25.1494, 13.8561) (25.3496, 14.0562) (25.3496, 14.303) knots 0 0 0 0 1 1 1 1
  line L4195 (24.9026, 13.8561) -> (25.1494, 13.8561) construction
  line L4196 (25.1494, 13.8561) -> (25.3496, 14.0562) construction
  line L4197 (25.3496, 14.0562) -> (25.3496, 14.303) construction
  spline S1324 degree 3 poles (17.3041, 5.4914) (17.3041, 5.7382) (17.1039, 5.9382) (16.8571, 5.9382) knots 0 0 0 0 1 1 1 1
  line L4198 (17.3041, 5.4914) -> (17.3041, 5.7382) construction
  line L4199 (17.3041, 5.7382) -> (17.1039, 5.9382) construction
  line L4200 (17.1039, 5.9382) -> (16.8571, 5.9382) construction
  spline S1325 degree 3 poles (16.8571, 5.9382) (16.6103, 5.9382) (16.4102, 5.7382) (16.4102, 5.4914) knots 0 0 0 0 1 1 1 1
  line L4201 (16.8571, 5.9382) -> (16.6103, 5.9382) construction
  line L4202 (16.6103, 5.9382) -> (16.4102, 5.7382) construction
  line L4203 (16.4102, 5.7382) -> (16.4102, 5.4914) construction
  spline S1326 degree 3 poles (16.4102, 5.4914) (16.4102, 5.2446) (16.6103, 5.0443) (16.8571, 5.0443) knots 0 0 0 0 1 1 1 1
  line L4204 (16.4102, 5.4914) -> (16.4102, 5.2446) construction
  line L4205 (16.4102, 5.2446) -> (16.6103, 5.0443) construction
  line L4206 (16.6103, 5.0443) -> (16.8571, 5.0443) construction
  spline S1327 degree 3 poles (16.8571, 5.0443) (17.1039, 5.0443) (17.3041, 5.2446) (17.3041, 5.4914) knots 0 0 0 0 1 1 1 1
  line L4207 (16.8571, 5.0443) -> (17.1039, 5.0443) construction
  line L4208 (17.1039, 5.0443) -> (17.3041, 5.2446) construction
  line L4209 (17.3041, 5.2446) -> (17.3041, 5.4914) construction
  spline S1328 degree 3 poles (14.75, 5.4914) (14.75, 5.7382) (14.5498, 5.9382) (14.303, 5.9382) knots 0 0 0 0 1 1 1 1
  line L4210 (14.75, 5.4914) -> (14.75, 5.7382) construction
  line L4211 (14.75, 5.7382) -> (14.5498, 5.9382) construction
  line L4212 (14.5498, 5.9382) -> (14.303, 5.9382) construction
  spline S1329 degree 3 poles (14.303, 5.9382) (14.0562, 5.9382) (13.8561, 5.7382) (13.8561, 5.4914) knots 0 0 0 0 1 1 1 1
  line L4213 (14.303, 5.9382) -> (14.0562, 5.9382) construction
  line L4214 (14.0562, 5.9382) -> (13.8561, 5.7382) construction
  line L4215 (13.8561, 5.7382) -> (13.8561, 5.4914) construction
  spline S1330 degree 3 poles (13.8561, 5.4914) (13.8561, 5.2446) (14.0562, 5.0443) (14.303, 5.0443) knots 0 0 0 0 1 1 1 1
  line L4216 (13.8561, 5.4914) -> (13.8561, 5.2446) construction
  line L4217 (13.8561, 5.2446) -> (14.0562, 5.0443) construction
  line L4218 (14.0562, 5.0443) -> (14.303, 5.0443) construction
  spline S1331 degree 3 poles (14.303, 5.0443) (14.5498, 5.0443) (14.75, 5.2446) (14.75, 5.4914) knots 0 0 0 0 1 1 1 1
  line L4219 (14.303, 5.0443) -> (14.5498, 5.0443) construction
  line L4220 (14.5498, 5.0443) -> (14.75, 5.2446) construction
  line L4221 (14.75, 5.2446) -> (14.75, 5.4914) construction
  spline S1332 degree 3 poles (17.3041, 8.0455) (17.3041, 8.2923) (17.1039, 8.4923) (16.8571, 8.4923) knots 0 0 0 0 1 1 1 1
  line L4222 (17.3041, 8.0455) -> (17.3041, 8.2923) construction
  line L4223 (17.3041, 8.2923) -> (17.1039, 8.4923) construction
  line L4224 (17.1039, 8.4923) -> (16.8571, 8.4923) construction
  spline S1333 degree 3 poles (16.8571, 8.4923) (16.6103, 8.4923) (16.4102, 8.2923) (16.4102, 8.0455) knots 0 0 0 0 1 1 1 1
  line L4225 (16.8571, 8.4923) -> (16.6103, 8.4923) construction
  line L4226 (16.6103, 8.4923) -> (16.4102, 8.2923) construction
  line L4227 (16.4102, 8.2923) -> (16.4102, 8.0455) construction
  spline S1334 degree 3 poles (16.4102, 8.0455) (16.4102, 7.7987) (16.6103, 7.5984) (16.8571, 7.5984) knots 0 0 0 0 1 1 1 1
  line L4228 (16.4102, 8.0455) -> (16.4102, 7.7987) construction
  line L4229 (16.4102, 7.7987) -> (16.6103, 7.5984) construction
  line L4230 (16.6103, 7.5984) -> (16.8571, 7.5984) construction
  spline S1335 degree 3 poles (16.8571, 7.5984) (17.1039, 7.5984) (17.3041, 7.7987) (17.3041, 8.0455) knots 0 0 0 0 1 1 1 1
  line L4231 (16.8571, 7.5984) -> (17.1039, 7.5984) construction
  line L4232 (17.1039, 7.5984) -> (17.3041, 7.7987) construction
  line L4233 (17.3041, 7.7987) -> (17.3041, 8.0455) construction
  spline S1336 degree 3 poles (17.3041, 10.5996) (17.3041, 10.8464) (17.1039, 11.0465) (16.8571, 11.0465) knots 0 0 0 0 1 1 1 1
  line L4234 (17.3041, 10.5996) -> (17.3041, 10.8464) construction
  line L4235 (17.3041, 10.8464) -> (17.1039, 11.0465) construction
  line L4236 (17.1039, 11.0465) -> (16.8571, 11.0465) construction
  spline S1337 degree 3 poles (16.8571, 11.0465) (16.6103, 11.0465) (16.4102, 10.8464) (16.4102, 10.5996) knots 0 0 0 0 1 1 1 1
  line L4237 (16.8571, 11.0465) -> (16.6103, 11.0465) construction
  line L4238 (16.6103, 11.0465) -> (16.4102, 10.8464) construction
  line L4239 (16.4102, 10.8464) -> (16.4102, 10.5996) construction
  spline S1338 degree 3 poles (16.4102, 10.5996) (16.4102, 10.3528) (16.6103, 10.1525) (16.8571, 10.1525) knots 0 0 0 0 1 1 1 1
  line L4240 (16.4102, 10.5996) -> (16.4102, 10.3528) construction
  line L4241 (16.4102, 10.3528) -> (16.6103, 10.1525) construction
  line L4242 (16.6103, 10.1525) -> (16.8571, 10.1525) construction
  spline S1339 degree 3 poles (16.8571, 10.1525) (17.1039, 10.1525) (17.3041, 10.3528) (17.3041, 10.5996) knots 0 0 0 0 1 1 1 1
  line L4243 (16.8571, 10.1525) -> (17.1039, 10.1525) construction
  line L4244 (17.1039, 10.1525) -> (17.3041, 10.3528) construction
  line L4245 (17.3041, 10.3528) -> (17.3041, 10.5996) construction
  spline S1340 degree 3 poles (17.3041, 13.1537) (17.3041, 13.4005) (17.1039, 13.6006) (16.8571, 13.6006) knots 0 0 0 0 1 1 1 1
  line L4246 (17.3041, 13.1537) -> (17.3041, 13.4005) construction
  line L4247 (17.3041, 13.4005) -> (17.1039, 13.6006) construction
  line L4248 (17.1039, 13.6006) -> (16.8571, 13.6006) construction
  spline S1341 degree 3 poles (16.8571, 13.6006) (16.6103, 13.6006) (16.4102, 13.4005) (16.4102, 13.1537) knots 0 0 0 0 1 1 1 1
  line L4249 (16.8571, 13.6006) -> (16.6103, 13.6006) construction
  line L4250 (16.6103, 13.6006) -> (16.4102, 13.4005) construction
  line L4251 (16.4102, 13.4005) -> (16.4102, 13.1537) construction
  spline S1342 degree 3 poles (16.4102, 13.1537) (16.4102, 12.9069) (16.6103, 12.7067) (16.8571, 12.7067) knots 0 0 0 0 1 1 1 1
  line L4252 (16.4102, 13.1537) -> (16.4102, 12.9069) construction
  line L4253 (16.4102, 12.9069) -> (16.6103, 12.7067) construction
  line L4254 (16.6103, 12.7067) -> (16.8571, 12.7067) construction
  spline S1343 degree 3 poles (16.8571, 12.7067) (17.1039, 12.7067) (17.3041, 12.9069) (17.3041, 13.1537) knots 0 0 0 0 1 1 1 1
  line L4255 (16.8571, 12.7067) -> (17.1039, 12.7067) construction
  line L4256 (17.1039, 12.7067) -> (17.3041, 12.9069) construction
  line L4257 (17.3041, 12.9069) -> (17.3041, 13.1537) construction
  spline S1344 degree 3 poles (17.3041, 15.7078) (17.3041, 15.9546) (17.1039, 16.1547) (16.8571, 16.1547) knots 0 0 0 0 1 1 1 1
  line L4258 (17.3041, 15.7078) -> (17.3041, 15.9546) construction
  line L4259 (17.3041, 15.9546) -> (17.1039, 16.1547) construction
  line L4260 (17.1039, 16.1547) -> (16.8571, 16.1547) construction
  spline S1345 degree 3 poles (16.8571, 16.1547) (16.6103, 16.1547) (16.4102, 15.9546) (16.4102, 15.7078) knots 0 0 0 0 1 1 1 1
  line L4261 (16.8571, 16.1547) -> (16.6103, 16.1547) construction
  line L4262 (16.6103, 16.1547) -> (16.4102, 15.9546) construction
  line L4263 (16.4102, 15.9546) -> (16.4102, 15.7078) construction
  spline S1346 degree 3 poles (16.4102, 15.7078) (16.4102, 15.461) (16.6103, 15.2608) (16.8571, 15.2608) knots 0 0 0 0 1 1 1 1
  line L4264 (16.4102, 15.7078) -> (16.4102, 15.461) construction
  line L4265 (16.4102, 15.461) -> (16.6103, 15.2608) construction
  line L4266 (16.6103, 15.2608) -> (16.8571, 15.2608) construction
  spline S1347 degree 3 poles (16.8571, 15.2608) (17.1039, 15.2608) (17.3041, 15.461) (17.3041, 15.7078) knots 0 0 0 0 1 1 1 1
  line L4267 (16.8571, 15.2608) -> (17.1039, 15.2608) construction
  line L4268 (17.1039, 15.2608) -> (17.3041, 15.461) construction
  line L4269 (17.3041, 15.461) -> (17.3041, 15.7078) construction
  spline S1348 degree 3 poles (17.3041, 18.2619) (17.3041, 18.5087) (17.1039, 18.7088) (16.8571, 18.7088) knots 0 0 0 0 1 1 1 1
  line L4270 (17.3041, 18.2619) -> (17.3041, 18.5087) construction
  line L4271 (17.3041, 18.5087) -> (17.1039, 18.7088) construction
  line L4272 (17.1039, 18.7088) -> (16.8571, 18.7088) construction
  spline S1349 degree 3 poles (16.8571, 18.7088) (16.6103, 18.7088) (16.4102, 18.5087) (16.4102, 18.2619) knots 0 0 0 0 1 1 1 1
  line L4273 (16.8571, 18.7088) -> (16.6103, 18.7088) construction
  line L4274 (16.6103, 18.7088) -> (16.4102, 18.5087) construction
  line L4275 (16.4102, 18.5087) -> (16.4102, 18.2619) construction
  spline S1350 degree 3 poles (16.4102, 18.2619) (16.4102, 18.0151) (16.6103, 17.8149) (16.8571, 17.8149) knots 0 0 0 0 1 1 1 1
  line L4276 (16.4102, 18.2619) -> (16.4102, 18.0151) construction
  line L4277 (16.4102, 18.0151) -> (16.6103, 17.8149) construction
  line L4278 (16.6103, 17.8149) -> (16.8571, 17.8149) construction
  spline S1351 degree 3 poles (16.8571, 17.8149) (17.1039, 17.8149) (17.3041, 18.0151) (17.3041, 18.2619) knots 0 0 0 0 1 1 1 1
  line L4279 (16.8571, 17.8149) -> (17.1039, 17.8149) construction
  line L4280 (17.1039, 17.8149) -> (17.3041, 18.0151) construction
  line L4281 (17.3041, 18.0151) -> (17.3041, 18.2619) construction
  spline S1352 degree 3 poles (17.3041, 20.816) (17.3041, 21.0628) (17.1039, 21.2629) (16.8571, 21.2629) knots 0 0 0 0 1 1 1 1
  line L4282 (17.3041, 20.816) -> (17.3041, 21.0628) construction
  line L4283 (17.3041, 21.0628) -> (17.1039, 21.2629) construction
  line L4284 (17.1039, 21.2629) -> (16.8571, 21.2629) construction
  spline S1353 degree 3 poles (16.8571, 21.2629) (16.6103, 21.2629) (16.4102, 21.0628) (16.4102, 20.816) knots 0 0 0 0 1 1 1 1
  line L4285 (16.8571, 21.2629) -> (16.6103, 21.2629) construction
  line L4286 (16.6103, 21.2629) -> (16.4102, 21.0628) construction
  line L4287 (16.4102, 21.0628) -> (16.4102, 20.816) construction
  spline S1354 degree 3 poles (16.4102, 20.816) (16.4102, 20.5692) (16.6103, 20.369) (16.8571, 20.369) knots 0 0 0 0 1 1 1 1
  line L4288 (16.4102, 20.816) -> (16.4102, 20.5692) construction
  line L4289 (16.4102, 20.5692) -> (16.6103, 20.369) construction
  line L4290 (16.6103, 20.369) -> (16.8571, 20.369) construction
  spline S1355 degree 3 poles (16.8571, 20.369) (17.1039, 20.369) (17.3041, 20.5692) (17.3041, 20.816) knots 0 0 0 0 1 1 1 1
  line L4291 (16.8571, 20.369) -> (17.1039, 20.369) construction
  line L4292 (17.1039, 20.369) -> (17.3041, 20.5692) construction
  line L4293 (17.3041, 20.5692) -> (17.3041, 20.816) construction
  spline S1356 degree 3 poles (19.8582, 13.1537) (19.8582, 13.4005) (19.658, 13.6006) (19.4112, 13.6006) knots 0 0 0 0 1 1 1 1
  line L4294 (19.8582, 13.1537) -> (19.8582, 13.4005) construction
  line L4295 (19.8582, 13.4005) -> (19.658, 13.6006) construction
  line L4296 (19.658, 13.6006) -> (19.4112, 13.6006) construction
  spline S1357 degree 3 poles (19.4112, 13.6006) (19.1644, 13.6006) (18.9643, 13.4005) (18.9643, 13.1537) knots 0 0 0 0 1 1 1 1
  line L4297 (19.4112, 13.6006) -> (19.1644, 13.6006) construction
  line L4298 (19.1644, 13.6006) -> (18.9643, 13.4005) construction
  line L4299 (18.9643, 13.4005) -> (18.9643, 13.1537) construction
  spline S1358 degree 3 poles (18.9643, 13.1537) (18.9643, 12.9069) (19.1644, 12.7067) (19.4112, 12.7067) knots 0 0 0 0 1 1 1 1
  line L4300 (18.9643, 13.1537) -> (18.9643, 12.9069) construction
  line L4301 (18.9643, 12.9069) -> (19.1644, 12.7067) construction
  line L4302 (19.1644, 12.7067) -> (19.4112, 12.7067) construction
  spline S1359 degree 3 poles (19.4112, 12.7067) (19.658, 12.7067) (19.8582, 12.9069) (19.8582, 13.1537) knots 0 0 0 0 1 1 1 1
  line L4303 (19.4112, 12.7067) -> (19.658, 12.7067) construction
  line L4304 (19.658, 12.7067) -> (19.8582, 12.9069) construction
  line L4305 (19.8582, 12.9069) -> (19.8582, 13.1537) construction
  spline S1360 degree 3 poles (19.8582, 15.7078) (19.8582, 15.9546) (19.658, 16.1547) (19.4112, 16.1547) knots 0 0 0 0 1 1 1 1
  line L4306 (19.8582, 15.7078) -> (19.8582, 15.9546) construction
  line L4307 (19.8582, 15.9546) -> (19.658, 16.1547) construction
  line L4308 (19.658, 16.1547) -> (19.4112, 16.1547) construction
  spline S1361 degree 3 poles (19.4112, 16.1547) (19.1644, 16.1547) (18.9643, 15.9546) (18.9643, 15.7078) knots 0 0 0 0 1 1 1 1
  line L4309 (19.4112, 16.1547) -> (19.1644, 16.1547) construction
  line L4310 (19.1644, 16.1547) -> (18.9643, 15.9546) construction
  line L4311 (18.9643, 15.9546) -> (18.9643, 15.7078) construction